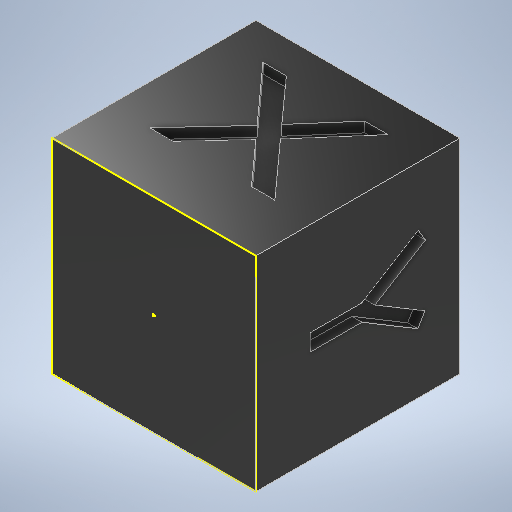
# Autodesk Inventor part: Cubo-001-001
Saved by Autodesk Inventor 2025.2 (Build 292293000, 293)
## iProperties
Created: 2025-01-25
Part Number: Cubo-001-001
Material: Steel, Carbon
Document SubType Name: Modeling
Designer: ishad
Density: 7.85 g/cm^3
Appearance: Glossy - Black
Author: ishad
## iProperties of the stored document Cubo-001-001_3DPrint.ipt
Created: 2025-01-25
Part Number: Cubo-001-001_3DPrint
Material: Generic
Document SubType Name: Modeling
Designer: ishad
Density: 1 g/cm^3
Appearance: Default
Author: ishad
Autodesk Inventor part; units mm, degrees
ref_plane "YZ Plane" through (0, 0, 0) normal (1, 0, 0) x (0, 1, 0)
ref_plane "XZ Plane" through (0, 0, 0) normal (0, 1, 0) x (-1, 0, 0)
ref_plane "XY Plane" through (0, 0, 0) normal (0, 0, 1) x (1, 0, 0)
sketch "Sketch1" plane through (0, 0, 0) normal (0, 0, 1) x (1, 0, 0)
  line L0 (10, -10.0138) -> (-10, -10.0138)
  line L1 (-10, -10.0138) -> (-10, 10.0138)
  line L2 (-10, 10.0138) -> (10, 10.0138)
  line L3 (10, 10.0138) -> (10, -10.0138)
  line L4 (10, -10.0138) -> (-10, 10.0138) construction
  line L5 (-10, -10.0138) -> (10, 10.0138) construction
  point P0 (0, 0)
  dimension "d0" = 20
  constraints: 12 end point, 2 midpoint, 2 parallel, 1 horizontal, 1 perpendicular
  measures "d0" distance of L1.end L2.end
extrude "Extrusion1" add sketch "Sketch1" along normal mid plane 20
sketch "Sketch2" plane through (0, 0, 10) normal (0, 0, 1) x (1, 0, 0)
  line L0 (10, 10.0138) -> (-10, 10.0138) projected
  line L1 (-10, 10.0138) -> (-10, -10.0138) projected
  line L2 (-10, -10.0138) -> (10, -10.0138) projected
  line L3 (10, -10.0138) -> (10, 10.0138) projected
  point P0 (0, 0)
sketch "Sketch3" plane through (-10, 10.0138, 10) normal (0, 1, 0) x (1, 0, 0)
  line L0 (10, 10) -> (3.9087, 16.7786)
  line L1 (3.9087, 16.7786) -> (6.1897, 16.7786)
  line L2 (6.1897, 16.7786) -> (11.262, 11.134)
  line L3 (11.262, 11.134) -> (16.1719, 5.6701)
  line L4 (16.1719, 5.6701) -> (13.8909, 5.6701)
  line L5 (13.8909, 5.6701) -> (10, 10)
  line L6 (11.262, 11.134) -> (16.1719, 16.7786)
  line L7 (16.1719, 16.7786) -> (13.8909, 16.7786)
  line L8 (13.8909, 16.7786) -> (10.1029, 12.4238)
  line L9 (3.9087, 5.6701) -> (8.981, 11.134)
  line L10 (10.1029, 9.8855) -> (6.1897, 5.6701)
  line L11 (6.1897, 5.6701) -> (3.9087, 5.6701)
  constraints: 24 end point, 5 point on line, 4 horizontal, 2 parallel
extrude "Extrusion2" cut sketch "Sketch3" against normal blind 1
sketch "Sketch4" plane through (0, 0, -10) normal (0, 0, -1) x (-1, 0, 0)
  line L0 (6.35, -6.35) -> (-6.35, -6.35)
  line L1 (-6.35, -6.35) -> (6.35, 6.35)
  line L2 (6.35, 6.35) -> (-6.35, 6.35)
  line L3 (6.35, -6.35) -> (6.35, -4.7625)
  line L4 (6.35, -4.7625) -> (-3.175, -4.7625)
  line L5 (-3.175, -4.7625) -> (6.35, 4.7625)
  line L6 (6.35, 4.7625) -> (-6.35, 4.7625)
  line L7 (6.35, 4.7625) -> (6.35, 6.35)
  line L8 (-6.35, 4.7625) -> (-6.35, 6.35)
  line L9 (-4.7625, -6.35) -> (-3.175, -4.7625)
  point P0 (0, 0)
  point P1 (4.7625, 4.7625)
  constraints: 20 end point, 3 parallel, 2 vertical, 1 point on line
extrude "Extrusion3" cut sketch "Sketch4" against normal blind 1
sketch "Sketch5" plane through (10, -10.0138, 10) normal (1, 0, 0) x (0, 0, -1)
  line L0 (5.3355, 9.1946) -> (5.3355, 10.8331)
  line L1 (5.3355, 10.8331) -> (10.3819, 10.8331)
  line L2 (10.3897, 9.1946) -> (5.3355, 9.1946)
  line L3 (10.3819, 10.8331) -> (15.9139, 14.2248)
  line L4 (15.9139, 14.2248) -> (16.6235, 13.0674)
  line L5 (16.6235, 13.0674) -> (11.6534, 10.0201)
  line L6 (11.6534, 10.0201) -> (16.5746, 7.0635)
  line L7 (16.5746, 7.0635) -> (15.875, 5.899)
  line L8 (15.875, 5.899) -> (10.3897, 9.1946)
  point P0 (10, 10.0138)
  point P1 (5.3355, 10.0138)
  constraints: 18 end point, 4 perpendicular, 1 horizontal, 1 midpoint, 1 vertical
extrude "Extrusion4" cut sketch "Sketch5" against normal blind 1
equation "\"d1\" = d0"
body "Solid1"
